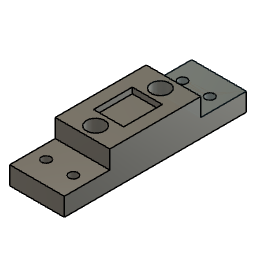
Accelerometer Base v4 (Autodesk Fusion 360 design; units mm, degrees)
Autodesk Fusion 360 part; units mm, degrees
sketch "Sketch1" plane through (0, 0, 0) normal (0, 1, 0) x (1, 0, 0)
  line L0 (-18.1, 70) -> (20, 70)
  line L1 (20, 70) -> (20, -57)
  line L2 (20, -57) -> (-18.1, -57)
  line L3 (-18.1, -57) -> (-18.1, 70)
  dimension "d1" = 127
  dimension "d2" = 38.1
  constraint horizontal L0
  constraint vertical L1
  constraint horizontal L2
  constraint vertical L3
  measures "d1" distance of L0.end L1.end
  measures "d2" distance of L1.end L2.end
extrude "Extrude1" add sketch "Sketch1" along normal blind 25.4
sketch "Sketch2" plane through (0, 25.4, 0) normal (0, 1, 0) x (-1, 0, 0)
  line L0 (18.1, 57) -> (-20, 57)
  line L1 (-20, 57) -> (-20, -70)
  line L2 (-20, -70) -> (18.1, -70)
  line L3 (18.1, -70) -> (18.1, 57)
  line L4 (18.1, 57) -> (-20, 57)
  line L5 (-20, 57) -> (-20, 25.25)
  line L6 (-20, 25.25) -> (18.1, 25.25)
  line L7 (18.1, 25.25) -> (18.1, 57)
  line L8 (18.1, -70) -> (-20, -70)
  line L9 (-20, -70) -> (-20, -38.25)
  line L10 (-20, -38.25) -> (18.1, -38.25)
  line L11 (18.1, -38.25) -> (18.1, -70)
  dimension "d5" = 31.75
  dimension "d6" = 31.75
  constraint horizontal L4
  constraint vertical L5
  constraint horizontal L6
  constraint vertical L7
  constraint coincident L0.start L3.end
  constraint horizontal L8
  constraint vertical L9
  constraint horizontal L10
  constraint vertical L11
  constraint coincident L1 L9.end
  constraint coincident L2.end L3.start
  measures "d5" distance of L0.start L6.end
  measures "d6" distance of L2.end L10.end
extrude "Extrude2" cut sketch "Sketch2" against normal blind 12.7 contours L0 L1 L3 L4 L5 L6 L7 | L1 L2 L3 L8 L9 L10 L11
sketch "Sketch3" plane through (0, 12.7, 0) normal (0, 1, 0) x (-1, 0, 0)
  line L0 (18.1, 25.25) -> (18.1, 57)
  line L1 (18.1, 57) -> (-20, 57)
  line L2 (-20, 57) -> (-20, 25.25)
  line L3 (-20, 25.25) -> (18.1, 25.25)
  circle A0 centre (8.575, 41.125) radius 3.175
  circle A1 centre (-10.475, 41.125) radius 3.175
  dimension "d9" = 6.35
  dimension "d10" = 15.875
  dimension "d12" = 6.35
  dimension "d13" = 15.875
  dimension "d15" = 19.05
  dimension "d16" = 9.525
  measures "d9" diameter of A0
  measures "d10" distance of L1 A0.centre
  measures "d12" diameter of A1
  measures "d13" distance of L1 A1.centre
  measures "d15" distance of A0.centre A1.centre
  measures "d16" distance of L2 A1.centre
extrude "Extrude3" cut sketch "Sketch3" against normal blind 30 contours A0 | A1
sketch "Sketch4" plane through (0, 12.7, 0) normal (0, 1, 0) x (-1, 0, 0)
  line L0 (18.1, -38.25) -> (-20, -38.25)
  line L1 (-20, -38.25) -> (-20, -70)
  line L2 (-20, -70) -> (18.1, -70)
  line L3 (18.1, -70) -> (18.1, -38.25)
sketch "Sketch5" plane through (0, 12.7, 0) normal (0, 1, 0) x (-1, 0, 0)
  circle A0 centre (-10.475, -54.125) radius 3.175
  circle A1 centre (8.575, -54.125) radius 3.175
  line L0 (-20, -38.25) -> (-20, -70)
  line L1 (-20, -70) -> (18.1, -70)
  dimension "d19" = 6.35
  dimension "d20" = 6.35
  dimension "d21" = 9.525
  dimension "d22" = 19.05
  dimension "d23" = 15.875
  dimension "d24" = 15.875
  measures "d19" diameter of A0
  measures "d20" diameter of A1
  measures "d21" distance of A0.centre L0
  measures "d22" distance of A0.centre A1.centre
  measures "d23" distance of A0.centre L1
  measures "d24" distance of A1.centre L1
extrude "Extrude4" cut sketch "Sketch5" against normal blind 40
sketch "Sketch6" plane through (0, 25.4, 0) normal (0, 1, 0) x (-1, 0, 0)
  line L0 (18.1, 25.25) -> (-20, 25.25)
  line L1 (-20, 25.25) -> (-20, -38.25)
  line L2 (-20, -38.25) -> (18.1, -38.25)
  line L3 (18.1, -38.25) -> (18.1, 25.25)
  line L4 (9.55, -20) -> (-11.45, -20)
  line L5 (-11.45, -20) -> (-11.45, 7)
  line L6 (-11.45, 7) -> (9.55, 7)
  line L7 (9.55, 7) -> (9.55, -20)
  circle A0 centre (-0.95, 16.125) radius 6.35
  circle A1 centre (-0.95, -29.125) radius 6.35
  dimension "d27" = 21
  dimension "d28" = 27
  dimension "d29" = 18.25
  dimension "d30" = 8.55
  dimension "d31" = 12.7
  dimension "d32" = 9.125
  dimension "d33" = 19.05
  dimension "d34" = 12.7
  dimension "d35" = 9.125
  dimension "d36" = 19.05
  constraint horizontal L4
  constraint vertical L5
  constraint horizontal L6
  constraint vertical L7
  measures "d27" distance of L4.start L4.end
  measures "d28" distance of L4.start L6.end
  measures "d29" distance of L2 L4
  measures "d30" distance of L1 L5
  measures "d31" diameter of A0
  measures "d32" distance of L0 A0.centre
  measures "d33" distance of L3 A0.centre
  measures "d34" diameter of A1
  measures "d35" distance of L2 A1.centre
  measures "d36" distance of L3 A1.centre
extrude "Extrude5" cut sketch "Sketch6" against normal blind 4 contours L4 L5 L6 L7 | A0 | A1
sketch "Sketch7" plane through (0, 25.4, 0) normal (0, 1, 0) x (-1, 0, 0)
  line L0 (-11.45, -20) -> (-11.45, 7)
  line L1 (-11.45, 7) -> (9.55, 7)
  line L2 (9.55, 7) -> (9.55, -20)
  line L3 (9.55, -20) -> (-11.45, -20)
  circle A0 centre (-0.95, 16.125) radius 6.35
  circle A1 centre (-0.95, -29.125) radius 6.35
  line L4 (18.1, 25.25) -> (-20, 25.25)
  line L5 (-20, 25.25) -> (-20, -38.25)
  line L6 (-20, -38.25) -> (18.1, -38.25)
  line L7 (18.1, -38.25) -> (18.1, 25.25)
  circle A2 centre (-0.95, -29.125) radius 6.35
  circle A3 centre (-0.95, 16.125) radius 6.35
  dimension "d39" = 12.7
  dimension "d40" = 12.7
  constraint concentric A1 A2
  constraint concentric A0 A3
  measures "d39" diameter of A2
  measures "d40" diameter of A3
extrude "Extrude6" cut sketch "Sketch7" against normal blind 12.7 contours A0 A3 | A1 A2
